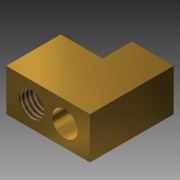
# Autodesk Inventor part: heHeaterBlock
Saved by Autodesk Inventor 2013 (Build 170138000, 138)
## iProperties
Created: 2015-01-15
Part Number: heHeaterBlock
Material: Generic
Document SubType Name: Modeling
Designer: dzban
Density: 1 g/cm^3
Author: dzban
Autodesk Inventor part; units mm, degrees
ref_plane "YZ Plane" through (0, 0, 0) normal (1, 0, 0) x (0, 1, 0)
ref_plane "XZ Plane" through (0, 0, 0) normal (0, 1, 0) x (-1, 0, 0)
ref_plane "XY Plane" through (0, 0, 0) normal (0, 0, 1) x (1, 0, 0)
sketch "Sketch1" plane through (0, 0, 0) normal (0, 0, 1) x (1, 0, 0)
  line L0 (0, 0) -> (0, 13)
  line L1 (0, 13) -> (10, 13)
  line L2 (10, 13) -> (10, 20)
  line L3 (10, 20) -> (20, 20)
  line L4 (20, 20) -> (20, 0)
  line L5 (20, 0) -> (0, 0)
  dimension "d0" = 20
  dimension "d2" = 20
  dimension "d3" = 10
  dimension "d4" = 7
  constraints: 12 end point, 3 horizontal, 3 vertical
  measures "d0" distance between parallel lines of L4 L0
  measures "d2" distance between parallel lines of L3 L5
  measures "d3" distance between parallel lines of L2 L0
  measures "d4" distance between parallel lines of L3 L1
extrude "Extrusion1" add sketch "Sketch1" along normal blind 10
sketch "Sketch2" plane through (0, 0, 0) normal (0, -1, 0) x (1, 0, 0)
  line L0 (20, 0) -> (20, 10) projected
  line L1 (0, 10) -> (20, 10) projected
  line L2 (0, 0) -> (0, 10) projected
  circle A0 centre (6, 5) radius 3
  circle A1 centre (14, 5) radius 3
  dimension "d7" = 6
  dimension "d9" = 6
  dimension "d10" = 5
  dimension "d11" = 6
  dimension "d12" = 6
  constraints: 2 centre point, 1 horizontal alignment
  measures "d7" diameter of A0
  measures "d9" distance from line of A0.centre L2
  measures "d10" distance from line of L1 A0.centre
  measures "d11" diameter of A1
  measures "d12" distance from line of L0 A1.centre
extrude "Extrusion2" cut sketch "Sketch2" against normal blind 22
sketch "Sketch3" plane through (0, 0, 0) normal (0, 0, -1) x (-1, 0, 0)
  line L0 (0, 0) -> (0, 13) projected
  line L1 (-20, 0) -> (0, 0) projected
  circle A0 centre (-10, 2.5) radius 1.25
  dimension "d15" = 2.5
  dimension "d17" = 2.5
  dimension "d18" = 10
  constraints: 1 centre point
  measures "d15" diameter of A0
  measures "d17" distance from line of A0.centre L1
  measures "d18" distance from line of L0 A0.centre
hole "Hole1" at (10, 2.5, 0) direction (0, 0, 1) diameter 2.5 depth 3 tip angle 118
thread "Thread1" size "M6x1" class "6H" standard "ANSI Metric M Profile" full length
body "Solid1"
